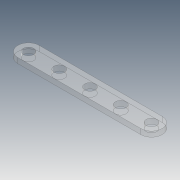
# Autodesk Inventor part: agregador-cilindros
Saved by Autodesk Inventor 2017 (Build 210142000, 142)
## iProperties
Created: 2018-08-15
Part Number: agregador-cilindros
Material: PMMA Plastic
Document SubType Name: Sheet Metal
Designer: Luiz Gustavo
Density: 1.188 g/cm^3
Sheet Metal Rule: Default_mm
Appearance: Polycarbonate - Clear
Author: Luiz Gustavo
Autodesk Inventor part; units mm, degrees
ref_plane "YZ Plane" through (0, 0, 0) normal (1, 0, 0) x (0, 1, 0)
ref_plane "XZ Plane" through (0, 0, 0) normal (0, 1, 0) x (-1, 0, 0)
ref_plane "XY Plane" through (0, 0, 0) normal (0, 0, 1) x (1, 0, 0)
sketch "Sketch1" plane through (0, 0, 0) normal (0, 0, 1) x (1, 0, 0)
  line L0 (-46.4, 0) -> (46.4, 0) construction
  line L1 (-46.4, 8) -> (46.4, 8)
  line L2 (46.4, -8) -> (-46.4, -8)
  arc A0 (-46.4, 8) -> (-46.4, -8) centre (-46.4, 0) ccw
  arc A1 (46.4, -8) -> (46.4, 8) centre (46.4, 0) ccw
  circle A2 centre (-46.4, 0) radius 4
  circle A3 centre (46.4, 0) radius 4
  circle A4 centre (0, 0) radius 4
  circle A5 centre (-23.2, 0) radius 4
  circle A6 centre (23.2, 0) radius 4
  dimension "d0" = 8
  dimension "d1" = 4
  dimension "d2" = 23.2
  dimension "d3" = 23.2
  dimension "d4" = 23.2
  measures "d0" diameter of A2
  measures "d1" radial gap between concentric circles of A0 A2
  measures "d2" distance of A5.centre point (0, 0)
  measures "d3" distance of L0.start A5.centre
  measures "d4" distance of A6.centre L0.end
extrude "Plate1" add sketch "Sketch1" along normal blind 4
equation "\"d3\" = d2"
equation "\"d4\" = d2"
equation "\"BendRadius\" = Thickness"
equation "\"BendReliefWidth\" = Thickness"
equation "\"BendReliefDepth\" = 0.5 * Thickness"
equation "\"CornerReliefSize\" = 4 * Thickness"
equation "\"MinimumRemnant\" = 2 * Thickness"
equation "\"TransitionRadius\" = BendRadius"
equation "\"JacobiRadiusSize\" = BendRadius"
equation "\"GapSize\" = Thickness"
equation "\"d5\" = BendRadius"
equation "\"Thickness\" = 4"
body "Solid1"
